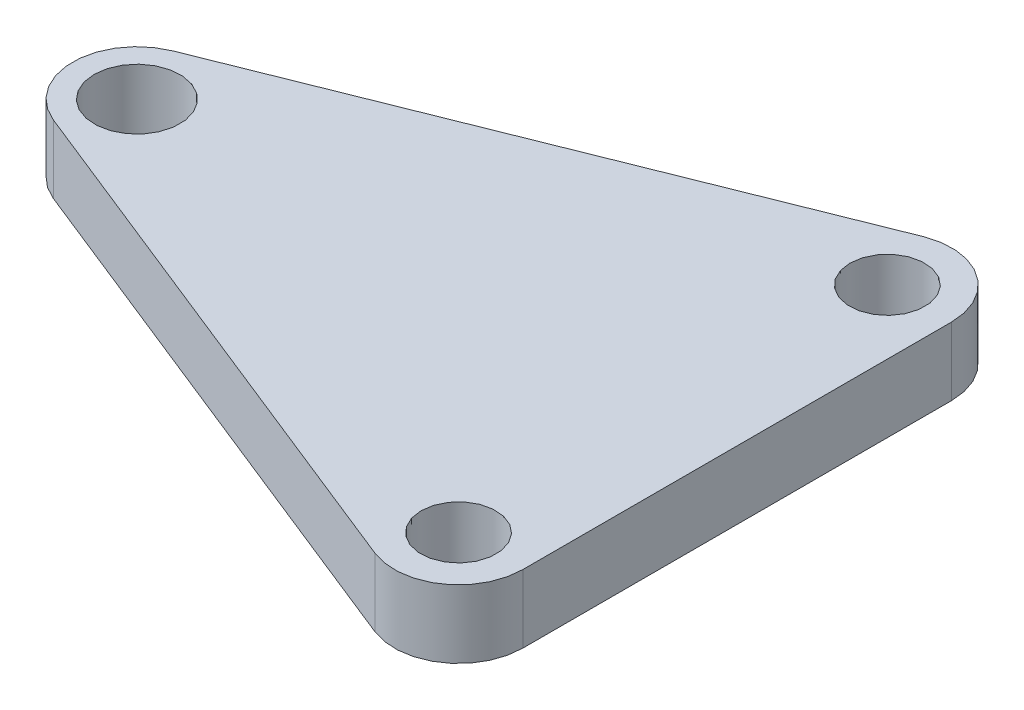
# Autodesk Inventor part: Cable Manegment
Saved by Autodesk Inventor 2023 (Build 270158000, 158)
## iProperties
Created: 2022-11-14
Part Number: Cable Manegment
Material: Generic
Document SubType Name: Modeling
Designer: deli
Density: 1 g/cm^3
Appearance: Default
Author: deli
Autodesk Inventor part; units mm, degrees
ref_plane "YZ Plane" through (0, 0, 0) normal (1, 0, 0) x (0, 1, 0)
ref_plane "XZ Plane" through (0, 0, 0) normal (0, 1, 0) x (-1, 0, 0)
ref_plane "XY Plane" through (0, 0, 0) normal (0, 0, 1) x (1, 0, 0)
sketch "Sketch1" plane through (0, 0, 0) normal (0, 1, 0) x (-1, 0, 0)
  circle A0 centre (17.9534, 95.7145) radius 1.75
  circle A1 centre (17.9534, 75.7145) radius 1.75
  arc A2 (19.0676, 98.4999) -> (14.9534, 95.7145) centre (17.9534, 95.7145) ccw
  arc A3 (14.9534, 75.7145) -> (19.0676, 72.9291) centre (17.9534, 75.7145) ccw
  arc A4 (44.0676, 82.9291) -> (44.0676, 88.4999) centre (42.9534, 85.7145) ccw
  circle A5 centre (42.9534, 85.7145) radius 2
  line L0 (19.0676, 98.4999) -> (44.0676, 88.4999)
  line L1 (14.9534, 95.7145) -> (14.9534, 75.7145)
  line L2 (19.0676, 72.9291) -> (44.0676, 82.9291)
  point P0 (0, 0)
  dimension "d0" = 3.5
  dimension "d1" = 6
  dimension "d2" = 4
  dimension "d3" = 20
  dimension "d4" = 25
  constraints: 6 centre point, 6 end point, 6 point on circle, 6 tangent, 3 coincident, 3 equal radius, 1 equal length, 1 vertical
  measures "d0" diameter of A0
  measures "d1" diameter of A2
  measures "d2" diameter of A5
  measures "d3" distance of L1.start L1.end
  measures "d4" horizontal distance of A0.centre A5.centre
extrude "Extrusion1" add sketch "Sketch1" along normal blind 3.175
body "Solid1"
